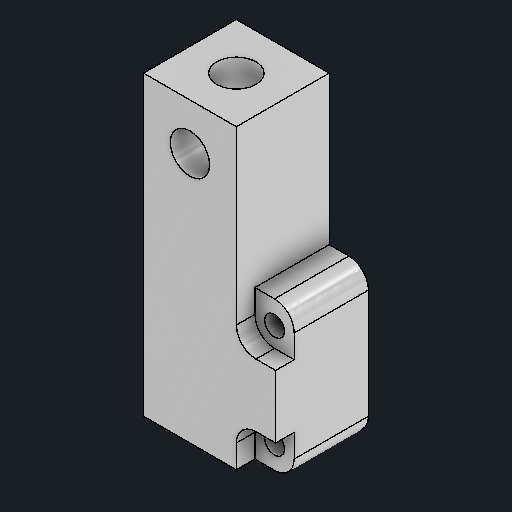
# Autodesk Inventor part: B Idler (Tulip)
Saved by Autodesk Inventor 2026.2 (Build 302298000, 298)
## iProperties
Created: 2025-04-15
Part Number: B Idler (Tulip)
Material: Aluminum 6061
Document SubType Name: Modeling
Designer: Joshua Eah
Density: 2.7 g/cm^3
Appearance: Machined - Aluminum
Author: Joshua Eah
Autodesk Inventor part; units mm, degrees
ref_plane "YZ Plane" through (0, 0, 0) normal (1, 0, 0) x (0, 1, 0)
ref_plane "XZ Plane" through (0, 0, 0) normal (0, 1, 0) x (-1, 0, 0)
ref_plane "XY Plane" through (0, 0, 0) normal (0, 0, 1) x (1, 0, 0)
sketch "Base Profile" plane through (0, 0, 0) normal (0, 1, 0) x (-1, 0, 0)
  line L0 (0, 0) -> (15, 0)
  line L1 (15, 0) -> (15, -15)
  line L2 (15, -15) -> (0, -15)
  line L3 (0, -15) -> (0, 0)
  line L4 (15, -15) -> (15, -21.35)
  line L5 (15, -21.35) -> (0, -21.35)
  line L6 (0, -21.35) -> (0, -15)
  dimension "d164" = 15
  dimension "d165" = 15
  dimension "d376" = 6.35
  constraints: 14 end point, 3 perpendicular, 2 parallel, 1 horizontal, 1 vertical
  measures "d164" distance of L1.end L2.end
  measures "d165" distance of L0.end L1.end
  measures "d376" distance of L1.end L4.end
extrude "Stock" add sketch "Base Profile" against normal blind 33
extrude "Extrusion Post" add sketch "Base Profile" along normal blind 15 contours L0 L1 L2 L3
sketch "Front Profile" plane through (0, -33, 0) normal (1, 0, 0) x (0, 0, -1)
  line L0 (0, 0) -> (0, 48) projected
  circle A0 centre (7.5, 40.5) radius 3.175
  line L1 (0, 48) -> (15, 48) projected
  line L2 (15, 33) -> (15, 48) projected
  line L3 (15, 33) -> (21.35, 33) projected
  line L4 (21.35, 33) -> (21.35, 0) projected
  line L5 (21.35, 0) -> (0, 0) projected
  line L6 (0, 7.5) -> (21.35, 7.5)
  line L7 (0, 16.5) -> (21.35, 16.5)
  line L8 (15, 33) -> (15, 0)
  line L9 (0, 24) -> (21.35, 24)
  line L10 (21.35, 24) -> (15, 16.5) construction
  line L11 (15, 0) -> (21.35, 7.5) construction
  circle A1 centre (18.175, 20.25) radius 1.5
  circle A2 centre (18.175, 3.75) radius 1.5
  circle A3 centre (18.175, 3.75) radius 3.175
  line L12 (21.35, 33) -> (21.35, 0) projected
  circle A4 centre (18.175, 20.25) radius 3.175
  line L13 (15, 20.25) -> (21.35, 20.25)
  line L14 (15, 3.75) -> (21.35, 3.75)
  line L15 (18.175, 17.075) -> (21.35, 17.075)
  line L16 (18.175, 6.925) -> (21.35, 6.925)
  point P0 (15, 24)
  point P1 (16.675, 3.75)
  point P2 (19.675, 3.75)
  point P3 (19.675, 20.25)
  point P4 (16.675, 20.25)
  dimension "d317" = 6.35
  dimension "d318" = 7.5
  dimension "d319" = 7.5
  dimension "d377" = 7.5
  dimension "d378" = 9
  dimension "d379" = 7.5
  dimension "d382" = 3
  dimension "d383" = 3
  constraints: 20 end point, 6 point on circle, 6 point on line, 5 centre point, 5 midpoint, 3 horizontal, 3 perpendicular, 3 tangent, 2 coincident, 6 other
  measures "d317" diameter of A0
  measures "d318" distance from line of A0.centre L0
  measures "d319" distance from line of A0.centre L1
  measures "d377" distance between parallel lines of L5 L6
  measures "d378" distance between parallel lines of L6 L7
  measures "d379" distance between parallel lines of L7 L9
  measures "d382" diameter of A1
  measures "d383" diameter of A2
extrude "Side Clearance" cut sketch "Front Profile" against normal through all contours L8 L3 L4 L9
hole "Front Mounting Hole" at (0, 7.5, -7.5) direction (-1, 0, 0) diameter 3.2004 end through all start extended yes counterbore diameter 6.35 counterbore depth 10.675 clearance for "Socket Head Cap Screw" size "M3" standard "Ansi Metric M Profile"
sketch "Sketch33" plane through (0, 15, 0) normal (0, 1, 0) x (1, 0, 0)
  line L0 (-15, 15) -> (-15, 0) projected
  line L1 (-15, 0) -> (0, 0) projected
  line L2 (0, 0) -> (0, 15) projected
  line L3 (0, 15) -> (-15, 15) projected
  circle A0 centre (-7.5, 7.5) radius 3.175
  dimension "d340" = 6.35
  dimension "d341" = 7.5
  dimension "d342" = 7.5
  constraints: 1 centre point
  measures "d340" diameter of A0
  measures "d341" distance from line of A0.centre L2
  measures "d342" distance from line of A0.centre L1
hole "Top Mounting Hole" at (-7.5, 15, -7.5) direction (0, -1, 0) diameter 3.2004 end through all start extended yes counterbore diameter 6.35 counterbore depth 13.675 clearance for "Socket Head Cap Screw" size "M3" standard "Ansi Metric M Profile"
hole "Tensioner Screw Holes" at (0, -12.75, -18.175) at (0, -29.25, -18.175) direction (-1, 0, 0) diameter 3.2004 end through all counterbore diameter 6.35 counterbore depth 2.9972 clearance for "Socket Head Cap Screw" size "M3" standard "Ansi Metric M Profile"
extrude "Counterbore Clearance" cut sketch "Front Profile" against normal up to surface (2.9972 mm away) contours L8 A3 L4 L5 | L14 A2 A3 | A3 L14 A2 | A3 L16 L4 | L14 A2 | A2 L14 | L9 L4 A4 L8 | L13 A1 A4 | A4 L13 A1 | L15 A4 L4 | L13 A1 | A1 L13
fillet "Fillet3" radius 3.175 2 edges at (-8.9986, -9, -21.35) (-8.9986, -33, -21.35)
equation "\"d164\" = extrusionWidth"
equation "\"d165\" = extrusionWidth"
equation "\"d168\" = extrusionOffset"
equation "\"extrusionWidth\" = 15"
equation "\"idlerLength\" = 17"
equation "\"bearingOffsetFromBottom\" = 7.5"
equation "\"extrusionOffset\" = 33"
equation "\"bearingStackHeight\" = 9"
equation "\"bearingSlotLength\" = 4"
equation "\"bearingClearance\" = 13"
equation "\"pinSupportLength\" = 2"
body "Solid2"
